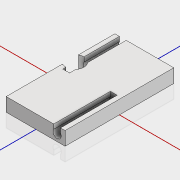
# Autodesk Inventor part: ЛЦМК.30000.10.00.01 Згт по одснование
Saved by Autodesk Inventor 2021.2 (Build 252289000, 289)
## iProperties
Created: 2025-11-22
Part Number: ЛЦМК.30000.10.00.01 Згт по одснование
Material: Типовые
Document SubType Name: Modeling
Designer: Захаров
Density: 1 g/cm^3
Appearance: По умолчанию
Author: Захаров
Autodesk Inventor part; units mm, degrees
ref_plane "YZ Plane" through (0, 0, 0) normal (1, 0, 0) x (0, 1, 0)
ref_plane "XZ Plane" through (0, 0, 0) normal (0, 1, 0) x (-1, 0, 0)
ref_plane "XY Plane" through (0, 0, 0) normal (0, 0, 1) x (1, 0, 0)
sketch "Эскиз1" plane through (0, 0, 0) normal (0, 1, 0) x (-1, 0, 0)
  line L0 (13, -24) -> (-13, -24)
  line L1 (-13, -24) -> (-13, 24)
  line L2 (-13, 24) -> (13, 24)
  line L3 (13, 24) -> (13, -24)
  line L4 (13, -24) -> (-13, 24) construction
  line L5 (-13, -24) -> (13, 24) construction
  point P0 (0, 0)
  dimension "d0" = 26
  dimension "d1" = 48
  constraints: 12 end point, 2 midpoint, 2 parallel, 1 horizontal, 1 perpendicular
  measures "d0" distance of L1.end L2.end
  measures "d1" distance of L0.end L1.end
extrude "Выдавливание1" add sketch "Эскиз1" along normal blind 6
sketch "Эскиз3" plane through (-13, 0, 24) normal (0, 0, 1) x (1, 0, 0)
  arc A0 (24, 4) -> (21, 4) centre (22.5, 3.005) ccw construction
  line L0 (26, 0) -> (26, 6) projected
  line L1 (21, 6) -> (24, 6)
  line L2 (24, 6) -> (24, 4)
  line L3 (24, 4) -> (21, 4) construction
  line L4 (21, 4) -> (21, 6)
  line L5 (21, 6) -> (24, 4) construction
  line L6 (24, 6) -> (21, 4) construction
  arc A1 (21, 4) -> (24, 4) centre (22.5, 3.005) ccw
  point P0 (13, 0)
  point P1 (22.5, 5)
  point P2 (22.5, 5)
  point P3 (22.5, 5)
  point P4 (22.5, 6)
  dimension "d8" = 3.6
  dimension "d10" = 2
  dimension "d11" = 3
  dimension "d12" = 2
  constraints: 12 end point, 5 midpoint, 4 point on circle, 2 centre point, 2 parallel, 1 horizontal, 1 horizontal alignment, 1 perpendicular, 1 vertical alignment
  measures "d8" diameter of A0
  measures "d10" distance of L1.end L2.end
  measures "d11" distance of L1.start L1.end
  measures "d12" distance from line of L0.end L2
extrude "Выдавливание3" cut sketch "Эскиз3" against normal blind 25
pattern_circular "Круговой массив1" count 2 over 360 about axis through (0, -10, 0) along (0, 1, 0) of "Выдавливание3"
sketch "Эскиз2" plane through (0, 6, 0) normal (0, 1, 0) x (1, 0, 0)
  circle A0 centre (-11.0356, 4.379) radius 4
  line L0 (13, 24) -> (-13, 24) projected
  point P0 (0, 0)
  dimension "d4" = 8
  constraints: 1 centre point
  measures "d4" diameter of A0
extrude "Выдавливание2" cut sketch "Эскиз2" against normal blind 6
sketch "Эскиз5" plane through (0, 6, 0) normal (0, 1, 0) x (1, 0, 0)
  line L0 (-13, 24) -> (-13, -24) projected
  arc A0 (-8, 1.7742) -> (-8, 6.9839) centre (-11.0356, 4.379) ccw projected
  arc A1 (-13, -4.1856) -> (-13.7446, 1.436) centre (-16.743, -1.8213) ccw
  arc A2 (-13, -6.1738) -> (-7.1165, 3.5787) centre (-23.7825, 6.9821) ccw
  point P0 (0, 0)
  point P1 (-5.684, 5.1513)
  point P2 (-13, 0.5431)
  constraints: 6 point on circle, 2 centre point, 2 point on line, 2 tangent
